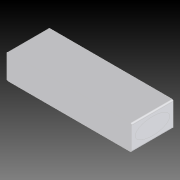
# Autodesk Inventor part: Turnigy 4S 5200 mah
Saved by Autodesk Inventor 2020 (Build 240168000, 168)
## iProperties
Created: 2015-05-07
Part Number: Turnigy 4S 5200 mah
Material: Типовой
Document SubType Name: Modeling
Designer: Tyler
Density: 1 g/cm^3
Appearance: По умолчанию
Mass: 194.33 g
Surface Area: 243.623 cm^2
Volume: 194.33 cm^3
Author: Tyler
Autodesk Inventor part; units mm, degrees
ref_plane "YZ Plane" through (0, 0, 0) normal (1, 0, 0) x (0, 1, 0)
ref_plane "XZ Plane" through (0, 0, 0) normal (0, 1, 0) x (-1, 0, 0)
ref_plane "XY Plane" through (0, 0, 0) normal (0, 0, 1) x (1, 0, 0)
sketch "Sketch1" plane through (0, 0, 0) normal (0, 1, 0) x (-1, 0, 0)
  line L0 (71.4375, 23.8125) -> (-71.4375, 23.8125)
  line L1 (-71.4375, 23.8125) -> (-71.4375, -23.8125)
  line L2 (-71.4375, -23.8125) -> (71.4375, -23.8125)
  line L3 (71.4375, -23.8125) -> (71.4375, 23.8125)
  point P0 (0, 0)
  point P1 (71.4375, 0)
  point P2 (0, -23.8125)
  dimension "d0" = 142.875
  dimension "d1" = 47.625
  constraints: 8 end point, 2 midpoint, 2 parallel, 1 horizontal, 1 horizontal alignment, 1 perpendicular, 1 vertical alignment
  measures "d0" distance of L2.end L1.end
  measures "d1" distance of L1.end L0.end
extrude "Extrusion1" add sketch "Sketch1" along normal blind 28.575
fillet "Fillet1" radius 1.5875 4 edges at (71.4375, 28.575, 0) (71.4375, 0, 0) (-71.4375, 0, 0) (-71.4375, 28.575, 0)
sketch "Sketch2" plane through (71.4375, 1.5875, -23.8125) normal (1, 0, 0) x (0, 0, -1)
  line L0 (0, 0) -> (-47.625, 0) projected
  line L1 (0, 0) -> (0, 25.4) projected
  line L2 (-47.625, 25.4) -> (0, 25.4) projected
  line L3 (-47.625, 0) -> (-47.625, 25.4) projected
  ellipse E0 centre (-23.8125, 12.7) end of major axis (-43.5575, 12.7) minor radius 9.5456
  point P0 (-23.8125, -1.5875)
  constraints: 2 other
sketch "Sketch3" plane through (-71.4375, 1.5875, -23.8125) normal (-1, 0, 0) x (0, 0, 1)
  line L0 (0, 25.4) -> (47.625, 25.4) projected
  line L1 (0, 0) -> (0, 25.4) projected
  line L2 (47.625, 0) -> (0, 0) projected
  line L3 (47.625, 0) -> (47.625, 25.4) projected
  ellipse E0 centre (23.8125, 12.7) end of major axis (2.3512, 12.7) minor radius 11.7224
  point P0 (23.8125, -1.5875)
  constraints: 2 other
extrude "Extrusion2" cut sketch "Sketch2" against normal blind 0.0025 contours E0
extrude "Extrusion3" cut sketch "Sketch3" against normal blind 0.0025 contours E0
body "Solid1"
